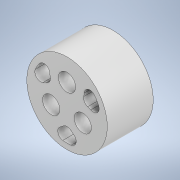
# Autodesk Inventor part: アーム 小さいカム
Saved by Autodesk Inventor 2020.2 (Build 242310000, 310)
## iProperties
Created: 2020-05-13
Part Number: アーム 小さいカム
Material: アルミニウム 2014-T6
Document SubType Name: Modeling
Designer: mozar
Density: 2.78927 g/cm^3
Appearance: サテン
Author: mozar
Autodesk Inventor part; units mm, degrees
ref_plane "YZ Plane" through (0, 0, 0) normal (1, 0, 0) x (0, 1, 0)
ref_plane "XZ Plane" through (0, 0, 0) normal (0, 1, 0) x (-1, 0, 0)
ref_plane "XY Plane" through (0, 0, 0) normal (0, 0, 1) x (1, 0, 0)
sketch "スケッチ1" plane through (0, 0, 0) normal (0, 0, 1) x (1, 0, 0)
  line L0 (0, 3.1754) -> (2.75, -1.5877)
  line L1 (2.75, -1.5877) -> (-2.75, -1.5877)
  line L2 (-2.75, -1.5877) -> (0, 3.1754)
  circle A0 centre (0, 3.1754) radius 1.5
  circle A1 centre (-2.75, -1.5877) radius 1.5
  circle A2 centre (2.75, -1.5877) radius 1.5
  circle A3 centre (0, 3.1754) radius 4
  circle A4 centre (-2.75, -1.5877) radius 4
  circle A5 centre (2.75, -1.5877) radius 4
  circle A6 centre (0, 0) radius 7.5
  circle A7 centre (0, 0) radius 4.6754
  circle A8 centre (0, 0) radius 7
  dimension "d0" = 3
  dimension "d1" = 3
  dimension "d2" = 3
  dimension "d3" = 2.5
  dimension "d4" = 2.5
  dimension "d5" = 2.5
  dimension "d6" = 15
  dimension "d7" = 2.8246
  dimension "d8" = 14
  dimension "d9" = 2.3246
  constraints: 9 centre point, 7 coincident, 6 end point, 2 tangent, 1 horizontal, 7 other
  measures "d0" diameter of A0
  measures "d1" diameter of A1
  measures "d2" diameter of A2
  measures "d3" radial gap between concentric circles of A0 A3
  measures "d4" radial gap between concentric circles of A1 A4
  measures "d5" radial gap between concentric circles of A2 A5
  measures "d6" diameter of A6
  measures "d7" radial gap between concentric circles of A6 A7
  measures "d8" diameter of A8
  measures "d9" radial gap between concentric circles of A8 A7
extrude "押し出し1" add sketch "スケッチ1" against normal blind 8 contours A5 A3 L0 | A5 A4 A0 | A0 A7 A3 A5 | L0 A3 A4 A5 | A4 A5 A3 L2 | A4 A3 A7 A0 | L2 A3 A4 | A3 A5 A7 A2 | A2 A4 A3 | A3 A7 A5 | A4 A3 A5 | A3 A5 A1 | A1 A7 A4 A3 | A7 A3 A8 | A4 A7 A3 | A4 A5 L1 | L1 A5 A3 A4 | A2 A7 A5 A4 | A3 A8 A5 A7 | A5 A8 A7 | A5 A4 A7 A1 | A7 A4 A8 | A7 A4 A8 A3 | A5 A7 A4 | A7 A5 A8 A4
sketch "スケッチ2" plane through (0, 0, 0) normal (0, 0, 1) x (1, 0, 0)
  circle A0 centre (0, 0) radius 7 projected
  circle A1 centre (2.75, -1.5877) radius 1.5 projected
  circle A2 centre (-2.75, -1.5877) radius 1.5 projected
  circle A3 centre (0, 3.1754) radius 1.5 projected
  circle A4 centre (0, 3.1754) radius 4
  circle A5 centre (-2.75, -1.5877) radius 4
  circle A6 centre (2.75, -1.5877) radius 4
  circle A7 centre (0, 0) radius 4.5
  dimension "d12" = 2.5
  dimension "d13" = 2.5
  dimension "d14" = 2.5
  dimension "d15" = 2.5
  constraints: 4 centre point
  measures "d12" radial gap between concentric circles of A3 A4
  measures "d13" radial gap between concentric circles of A2 A5
  measures "d14" radial gap between concentric circles of A1 A6
  measures "d15" radial gap between concentric circles of A0 A7
sketch "スケッチ3" plane through (0, 0, 0) normal (0, 0, 1) x (1, 0, 0)
  circle A0 centre (0, 3.1754) radius 1.5 projected
  circle A1 centre (-2.75, -1.5877) radius 1.5 projected
  circle A2 centre (2.75, -1.5877) radius 1.5 projected
  circle A3 centre (0, 0) radius 7 projected
  circle A4 centre (0, 3.1754) radius 3
  circle A5 centre (-2.75, -1.5877) radius 3
  circle A6 centre (2.75, -1.5877) radius 3
  circle A7 centre (0, 0) radius 7 projected
  circle A8 centre (0, 0) radius 6
  point P0 (-4.3667, -4.1148)
  point P1 (4.3667, -4.1148)
  point P2 (0, -2.7867)
  point P3 (5.7469, -1.7243)
  point P4 (1.3801, 5.8391)
  point P5 (2.4133, 1.3933)
  point P6 (-1.3801, 5.8391)
  point P7 (-5.7469, -1.7243)
  point P8 (-2.4133, 1.3933)
  dimension "d17" = 1
  dimension "d19" = 1.5
  dimension "d20" = 1.5
  dimension "d21" = 1.5
  constraints: 4 centre point, 2 coincident
  measures "d17" radial gap between concentric circles of A3 A8
  measures "d19" radial gap between concentric circles of A1 A5
  measures "d20" radial gap between concentric circles of A4 A0
  measures "d21" radial gap between concentric circles of A2 A6
extrude "押し出し2" cut sketch "スケッチ3" against normal blind 10 contours A4 A8 A6 | A4 A5 A8 | A5 A6 A8
fillet "フィレット1" radius 1 9 edges at (-1.3801, 5.8391, -4) (1.3801, 5.8391, -4) (5.7469, -1.7243, -4) (2.4133, 1.3933, -4) (-2.4133, 1.3933, -4) (-5.7469, -1.7243, -4) (-4.3667, -4.1148, -4) (0, -2.7867, -4) (4.3667, -4.1148, -4)
equation "\"d3\" = d4"
equation "\"d5\" = d4"
equation "\"d20\" = d19"
equation "\"d21\" = d19"
